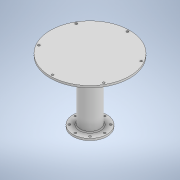
# Autodesk Inventor part: Connection_link_1
Saved by Autodesk Inventor 2021 (Build 250183000, 183)
## iProperties
Created: 2020-05-19
Part Number: Connection_link_1
Material: Generic
Document SubType Name: Modeling
Designer: Motius
Density: 1 g/cm^3
Appearance: Default
Author: Motius
Autodesk Inventor part; units mm, degrees
note: some values were not read from the file. Chosen so that the rebuilt part matches the saved one: direction of "Hole3".
ref_plane "YZ Plane" through (0, 0, 0) normal (1, 0, 0) x (0, 1, 0)
ref_plane "XZ Plane" through (0, 0, 0) normal (0, 1, 0) x (-1, 0, 0)
ref_plane "XY Plane" through (0, 0, 0) normal (0, 0, 1) x (1, 0, 0)
sketch "Sketch1" plane through (0, 0, 0) normal (0, 0, 1) x (1, 0, 0)
  line L0 (0, 91.7) -> (0, -91.7) construction
  line L1 (-16.3, 0) -> (97.8, 0) construction
  line L2 (0, -65.5) -> (0, 65.5)
  line L3 (0, -65.5) -> (81.5, -65.5)
  line L4 (81.5, -65.5) -> (81.5, 65.5)
  line L5 (81.5, 65.5) -> (0, 65.5)
  point P0 (0, 0)
  dimension "d2" = 131
  dimension "d12" = 81.5
  constraints: 8 end point, 1 collinear, 1 perpendicular, 1 vertical, 1 other
  measures "d2" distance of L3.end L4.end
  measures "d12" distance between parallel lines of L4 L0
revolve "Revolution1" add sketch "Sketch1" angle 360 about axis through (0, 0, 0) along (0, -1, 0)
sketch "Sketch4" plane through (0, 0, 0) normal (0, 0, 1) x (1, 0, 0)
  line L0 (-81.5, 65.5) -> (81.5, 65.5) construction
  line L1 (-81.5, -65.5) -> (81.5, -65.5) construction
  line L2 (0, 91) -> (0, -91) construction
  line L3 (-114.1, 0) -> (114.1, 0) construction
  line L4 (35, -61.5) -> (22, -61.5)
  line L5 (20, -59.5) -> (20, 56.5)
  line L6 (25, 61.5) -> (81.5, 61.5)
  line L7 (81.5, 65.5) -> (81.5, -65.5) construction
  line L8 (81.5, -65.5) -> (81.5, 61.5)
  arc A0 (20, -59.5) -> (22, -61.5) centre (22, -59.5) ccw
  arc A1 (25, 61.5) -> (20, 56.5) centre (25, 56.5) ccw
  line L9 (35, -65.5) -> (35, -61.5)
  line L10 (-81.5, -65.5) -> (81.5, -65.5) construction
  line L11 (35, -65.5) -> (81.5, -65.5)
  point P0 (0, 0)
  dimension "d35" = 20
  dimension "d36" = 4
  dimension "d37" = 2
  dimension "d39" = 35
  dimension "d40" = 5
  constraints: 12 end point, 4 point on circle, 4 tangent, 3 perpendicular, 3 point on line, 2 centre point, 2 collinear, 1 horizontal, 1 other
  measures "d35" distance between parallel lines of L2 L5
  measures "d36" distance between parallel lines of L1 L4
  measures "d37" radius of A0
  measures "d39" distance between parallel lines of L2 L9
  measures "d40" radius of A1
revolve "Revolution2" cut sketch "Sketch4" angle 360 about axis through (0, 0, 0) along (0, -1, 0)
sketch "Sketch2" plane through (0, -65.5, 0) normal (0, -1, 0) x (1, 0, 0)
  circle A0 centre (0, 0) radius 81.5 construction
  line L0 (-114.1, 0) -> (114.1, 0) construction
  line L1 (0, 114.1) -> (0, -114.1) construction
  circle A1 centre (0, 0) radius 21.25 construction
  circle A2 centre (0, 0) radius 30 construction
  point P0 (0, 30)
  point P1 (0, 21.25)
  point P2 (-21.2132, 21.2132)
  point P3 (-15.026, 15.026)
  point P4 (-30, 0)
  point P5 (-21.25, 0)
  point P6 (-21.2132, -21.2132)
  point P7 (-15.026, -15.026)
  point P8 (0, -30)
  point P9 (0, -21.25)
  point P10 (21.2132, -21.2132)
  point P11 (15.026, -15.026)
  point P12 (30, 0)
  point P13 (21.25, 0)
  point P14 (21.2132, 21.2132)
  point P15 (15.026, 15.026)
  point P16 (-4.5183, 21.1087)
  dimension "d6" = 42.5
  dimension "d7" = 60
  dimension "d10" = 360
  constraints: 2 coincident, 2 point on line, 2 vertical alignment, 21 other
hole "Hole2" at (0, -65.5, 30) at (-21.2132, -65.5, 21.2132) at (-30, -65.5, 0) at (-21.2132, -65.5, -21.2132) at (0, -65.5, -30) at (21.2132, -65.5, -21.2132) at (30, -65.5, 0) at (21.2132, -65.5, 21.2132) direction (0, 1, 0) diameter 4.5 depth 4 clearance for "Socket Head Cap Screw" size "M4" standard "Ansi Metric M Profile"
sketch "Sketch5" plane through (0, 65.5, 0) normal (0, 1, 0) x (1, 0, 0)
  line L0 (0, 114.1) -> (0, -114.1) construction
  line L1 (114.1, 0) -> (-114.1, 0) construction
  circle A0 centre (0, 0) radius 77 construction
  point P0 (0, 77)
  point P1 (-66.684, 38.5)
  point P2 (-66.684, -38.5)
  point P3 (0, -77)
  point P4 (66.684, -38.5)
  point P5 (66.684, 38.5)
  dimension "d45" = 154
  dimension "d43" = 360
  constraints: 1 coincident, 1 point on line, 1 vertical alignment, 9 other
hole "Hole3" at (0, 65.5, -77) at (-66.684, 65.5, -38.5) at (-66.684, 65.5, 38.5) at (0, 65.5, 77) at (66.684, 65.5, 38.5) at (66.684, 65.5, -38.5) direction (0, -1, 0) diameter 4.5 depth 4 clearance for "Socket Head Cap Screw" size "M4" standard "Ansi Metric M Profile"
body "Solid1"
